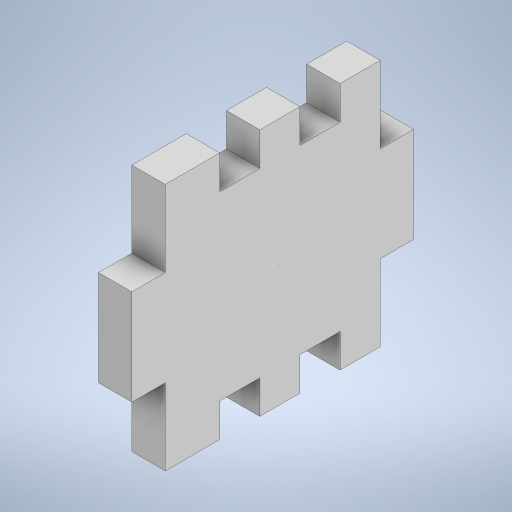
# Autodesk Inventor part: Stran Stran
Saved by Autodesk Inventor 2023 (Build 270158000, 158)
## iProperties
Created: 2022-12-19
Part Number: Stran Stran
Material: Generic
Document SubType Name: Modeling
Designer: David Zindović
Density: 1 g/cm^3
Appearance: Default
Author: David Zindović
Autodesk Inventor part; units mm, degrees
ref_plane "YZ Plane" through (0, 0, 0) normal (1, 0, 0) x (0, 1, 0)
ref_plane "XZ Plane" through (0, 0, 0) normal (0, 1, 0) x (-1, 0, 0)
ref_plane "XY Plane" through (0, 0, 0) normal (0, 0, 1) x (1, 0, 0)
sketch "Sketch1" plane through (0, 0, 0) normal (1, 0, 0) x (0, 1, 0)
  line L0 (13, -14.75) -> (-13, -14.75)
  line L1 (-13, -14.75) -> (-13, 14.75) construction
  line L2 (-13, 14.75) -> (13, 14.75)
  line L3 (13, 14.75) -> (13, -14.75)
  line L4 (5, -14.75) -> (-5, -14.75)
  line L5 (-5, -14.75) -> (-5, -11.25)
  line L6 (-5, -11.25) -> (5, -11.25)
  line L7 (5, -11.25) -> (5, -14.75)
  line L8 (-5, -11.25) -> (-13, -11.25)
  line L9 (-13, -11.25) -> (-13, -7.05)
  line L10 (-13, -7.05) -> (-9.5, -7.05)
  line L11 (-9.5, -7.05) -> (-9.5, -2.85)
  line L12 (-9.5, -2.85) -> (-13, -2.85)
  line L13 (-13, -2.85) -> (-13, 1.35)
  line L14 (-13, 1.35) -> (-9.5, 1.35)
  line L15 (-9.5, 1.35) -> (-9.5, 5.55)
  line L16 (-9.5, 5.55) -> (-13, 5.55)
  line L17 (5, 14.75) -> (-5, 14.75)
  line L18 (-5, 14.75) -> (-5, 11.25)
  line L19 (-5, 11.25) -> (5, 11.25)
  line L20 (5, 11.25) -> (5, 14.75)
  line L21 (-5, 11.25) -> (-13, 11.25)
  line L22 (0, 0) -> (0, -1.9359)
  line L23 (5, -11.25) -> (13, -11.25)
  line L24 (13, -7.05) -> (9.5, -7.05)
  line L25 (9.5, -7.05) -> (9.5, -2.85)
  line L26 (9.5, -2.85) -> (13, -2.85)
  line L27 (13, 1.35) -> (9.5, 1.35)
  line L28 (9.5, 1.35) -> (9.5, 5.55)
  line L29 (9.5, 5.55) -> (13, 5.55)
  line L30 (5, 11.25) -> (13, 11.25)
  line L31 (-13, 11.25) -> (-13, 5.55)
  line L32 (-13, 1.35) -> (-13, -2.85)
  line L33 (-13, -7.05) -> (-13, -11.25)
  point P0 (0, -14.75)
  point P1 (-13, 0)
  point P2 (0, -11.25)
  point P3 (-5, -14.75)
  dimension "d0" = 26
  dimension "d1" = 29.5
  dimension "d2" = 10
  dimension "d3" = 3.5
  dimension "d4" = 4.2
  dimension "d5" = 3.5
  dimension "d6" = 4.2
  dimension "d7" = 4.2
  dimension "d8" = 4.2
  dimension "d9" = 3.5
  constraints: 66 end point, 10 symmetric about line, 9 horizontal, 6 point on line, 5 parallel, 4 perpendicular, 4 vertical, 2 midpoint, 2 vertical alignment, 1 collinear, 1 horizontal alignment, 10 other
  measures "d0" distance of L0.start L0.end
  measures "d1" distance of L0.end L2.start
  measures "d2" distance of L5.end L6.end
  measures "d3" distance of L4.end L5.end
  measures "d4" distance of L8.end L9.end
  measures "d5" distance of L9.end L10.end
  measures "d6" distance of L10.end L11.end
  measures "d7" distance of L12.end L13.end
  measures "d8" distance of L14.end L15.end
  measures "d9" distance of L18.end L17.end
extrude "Extrusion1" add sketch "Sketch1" along normal mid plane 3.5 contours L0 L5 L6 L7 | L23 L6 L8 L9 L10 L11 L12 L13 L14 L15 L16 L31 L21 L19 L30 L3 L29 L28 L27 L26 L25 L24 | L19 L18 L2 L20
sketch "Sketch2" plane through (1.75, 0, 0) normal (1, 0, 0) x (0, 0, -1)
  point P0 (0, 0)
body "Solid1"
